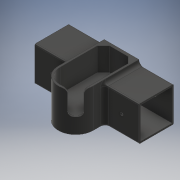
# Autodesk Inventor part: actuator_holder
Saved by Autodesk Inventor 2019.4 (Build 234330000, 330)
## iProperties
Created: 2020-10-05
Part Number: actuator_holder
Material: Generic
Document SubType Name: Modeling
Designer: deanv
Density: 1 g/cm^3
Appearance: Smooth - Black
Author: deanv
Autodesk Inventor part; units mm, degrees
ref_plane "YZ Plane" through (0, 0, 0) normal (1, 0, 0) x (0, 1, 0)
ref_plane "XZ Plane" through (0, 0, 0) normal (0, 1, 0) x (-1, 0, 0)
ref_plane "XY Plane" through (0, 0, 0) normal (0, 0, 1) x (1, 0, 0)
sketch "Sketch1" plane through (0, 0, 0) normal (0, 0, 1) x (1, 0, 0)
  line L0 (20, -37.4) -> (-20, -37.4) construction
  line L1 (-20, -37.4) -> (-20, 37.4) construction
  line L2 (-20, 37.4) -> (20, 37.4) construction
  line L3 (20, 37.4) -> (20, -37.4) construction
  line L4 (20, -37.4) -> (-20, 37.4) construction
  line L5 (-20, -37.4) -> (20, 37.4) construction
  line L6 (22.5, -39.9) -> (-22.5, -39.9) construction
  line L7 (-22.5, -39.9) -> (-22.5, 39.9) construction
  line L8 (-22.5, 39.9) -> (22.5, 39.9) construction
  line L9 (22.5, 39.9) -> (22.5, -39.9) construction
  line L10 (22.5, -39.9) -> (-22.5, 39.9) construction
  line L11 (-22.5, -39.9) -> (22.5, 39.9) construction
  line L12 (8.75, 10.75) -> (-8.75, 10.75)
  line L13 (-8.75, 10.75) -> (-8.75, 28.25)
  line L14 (-8.75, 28.25) -> (8.75, 28.25)
  line L15 (8.75, 28.25) -> (8.75, 10.75)
  line L16 (8.75, 10.75) -> (-8.75, 28.25) construction
  line L17 (-8.75, 10.75) -> (8.75, 28.25) construction
  line L18 (0, 39.9) -> (0, -39.9) construction
  line L19 (-22.5, 0) -> (22.5, 0) construction
  line L20 (-20, -17.4) -> (20, -17.4) construction
  line L21 (-20, 37.4) -> (20, 37.4)
  line L22 (20, 37.4) -> (20, -37.4)
  line L23 (20, -37.4) -> (-20, -37.4)
  line L24 (-20, -37.4) -> (-20, 37.4)
  line L25 (-22.5, -39.9) -> (22.5, -39.9)
  line L26 (22.5, -39.9) -> (22.5, 39.9)
  line L27 (22.5, 39.9) -> (-22.5, 39.9)
  line L28 (-22.5, 39.9) -> (-22.5, -39.9)
  line L29 (22.5, -0.5) -> (-22.5, -0.5) construction
  line L30 (-22.5, -0.5) -> (-22.5, 39.5) construction
  line L31 (-22.5, 39.5) -> (22.5, 39.5) construction
  line L32 (22.5, 39.5) -> (22.5, -0.5) construction
  line L33 (22.5, -0.5) -> (-22.5, 39.5) construction
  line L34 (-22.5, -0.5) -> (22.5, 39.5) construction
  line L35 (-22.5, 39.5) -> (22.5, 39.5)
  line L36 (22.5, 39.5) -> (22.5, 42)
  line L37 (22.5, 42) -> (-22.5, 42)
  line L38 (-22.5, 42) -> (-22.5, 39.5)
  line L39 (-22.5, -0.5) -> (22.5, -0.5)
  line L40 (22.5, -0.5) -> (22.5, -3)
  line L41 (22.5, -3) -> (-22.5, -3)
  line L42 (-22.5, -3) -> (-22.5, -0.5)
  line L43 (22.5, -39.9) -> (0, -17.4) construction
  line L44 (0, -39.9) -> (22.5, -17.4) construction
  line L45 (5.3033, -12.0967) -> (27.8033, -34.5967)
  line L46 (27.8033, -34.5967) -> (17.1967, -45.2033)
  line L47 (17.1967, -45.2033) -> (-5.3033, -22.7033)
  line L48 (-5.3033, -22.7033) -> (5.3033, -12.0967)
  line L49 (5.3033, -12.0967) -> (17.1967, -45.2033) construction
  line L50 (27.8033, -34.5967) -> (-5.3033, -22.7033) construction
  point P0 (0, 0)
  point P1 (0, 19.5)
  point P2 (0, 19.5)
  point P3 (11.25, -28.65)
  dimension "d0" = 40
  dimension "d1" = 74.8
  dimension "d2" = 79.8
  dimension "d3" = 45
  dimension "d4" = 17.5
  dimension "d5" = 17.5
  dimension "d6" = 20.4
  dimension "d7" = 20
  dimension "d12" = 40
  dimension "d13" = 2.5
  dimension "d14" = 2.5
  dimension "d78" = 22.5
  dimension "d79" = 15
  dimension "d80" = 22.5
  constraints: 102 end point, 20 parallel, 17 midpoint, 9 perpendicular, 8 horizontal, 6 point on line
  measures "d0" distance of L1.end L2.end
  measures "d1" distance of L0.end L1.end
  measures "d2" distance of L6.end L7.end
  measures "d3" distance of L7.end L8.end
  measures "d4" distance of L13.end L14.end
  measures "d5" distance between parallel lines of L14 L12
  measures "d6" distance from line of L8 point (0, 19.5)
  measures "d7" distance between parallel lines of L0 L20
  measures "d12" distance of L29.end L30.end
  measures "d13" distance of L36.end L35.end
  measures "d14" distance of L39.end L40.end
  measures "d78" horizontal distance of L18.end L44.end
  measures "d79" distance of L45.end L46.end
  measures "d80" horizontal distance of L45.start L45.end
extrude "Extrusion1" add sketch "Sketch1" along normal blind 20 contours L21 L22 L39 L24 | L39 L22 L41 L24 | L41 L22 L45 L48 L47 L23 L24 | L22 L23 L47 L48 L45
extrude "Extrusion2" add sketch "Sketch1" along normal blind 50 contours L24 L39 L28 L35 L26 L22 L21 | L24 L41 L28 L39 | L39 L26 L41 L22 | L24 L23 L47 L25 L28 L41 | L41 L26 L45 L22 | L28 L27 L26 L35 | L45 L26 L25 L47 L23 L22
extrude "Extrusion4" add sketch "Sketch1" along normal blind 50 contours L28 L27 L26 L35 | L38 L37 L36 L27
sketch "Sketch2" plane through (8.75, 10.75, 0) normal (-1, 0, 0) x (0, 0, 1)
  line L0 (0, 17.5) -> (20, 17.5) construction
  line L1 (20, 17.5) -> (20, 0) construction
  line L2 (20, 0) -> (0, 0) construction
  line L3 (0, 0) -> (0, 17.5) construction
  line L4 (20, 17.5) -> (10, 17.5) construction
  line L5 (10, 17.5) -> (10, 8.75) construction
  line L6 (10, 8.75) -> (20, 8.75) construction
  line L7 (20, 8.75) -> (20, 17.5) construction
  line L8 (10, 12.75) -> (10, 4.75) construction
  line L9 (6, 12.75) -> (6, 4.75)
  line L10 (14, 4.75) -> (14, 12.75)
  arc A0 (14, 12.75) -> (6, 12.75) centre (10, 12.75) ccw
  arc A1 (6, 4.75) -> (14, 4.75) centre (10, 4.75) ccw
  line L11 (10, 8.75) -> (18, 8.75) construction
  point P0 (0, -10.75)
  dimension "d19" = 10
  dimension "d20" = 8.75
  dimension "d96" = 4
  dimension "d97" = 90
  dimension "d98" = 8
  constraints: 26 end point, 5 parallel, 4 point on circle, 4 tangent, 3 horizontal, 3 perpendicular, 2 centre point, 1 coincident, 1 midpoint, 1 vertical
  measures "d19" distance of L6.end L5.end
  measures "d20" distance of L5.end L4.end
  measures "d96" distance of L11.start L8.end
  measures "d97" angle of L8 L11
  measures "d98" diameter of A1
fillet "Fillet1" radius 20 2 edges at (20, -37.4, 35) (-20, -37.4, 35)
fillet "Fillet2" radius 22.5 2 edges at (-22.5, -39.9, 25) (22.5, -39.9, 25)
sketch "Sketch4" plane through (22.5, 42, 50) normal (1, 0, 0) x (0, 0, -1)
  line L0 (50, 0) -> (0, 0) projected
  circle A0 centre (40, -22.5) radius 3 projected
  line L1 (30, -45) -> (50, -45) construction
  line L2 (50, -45) -> (50, 0) construction
  line L3 (50, 0) -> (30, 0) construction
  line L4 (30, 0) -> (30, -45) construction
  line L5 (30, -45) -> (50, 0) construction
  line L6 (50, -45) -> (30, 0) construction
  line L7 (50, -45) -> (5, -45)
  line L8 (5, -45) -> (5, 0)
  line L9 (5, 0) -> (50, 0)
  line L10 (50, 0) -> (50, -45)
  line L11 (5, -45) -> (50, 0) construction
  line L12 (50, -45) -> (5, 0) construction
  line L13 (48, -2) -> (7, -2)
  line L14 (7, -2) -> (7, -43)
  line L15 (7, -43) -> (48, -43)
  line L16 (48, -43) -> (48, -2)
  line L17 (48, -2) -> (7, -43) construction
  line L18 (7, -2) -> (48, -43) construction
  point P0 (50, -42)
  point P1 (27.5, -22.5)
  dimension "d42" = 45
  dimension "d43" = 45
  dimension "d44" = 41
  dimension "d45" = 41
  constraints: 36 end point, 6 parallel, 5 midpoint, 3 horizontal, 3 perpendicular, 1 point on line
  measures "d42" distance of L0.start L1.end
  measures "d43" distance of L8.end L9.end
  measures "d44" distance of L15.end L14.end
  measures "d45" distance of L14.end L13.end
extrude "Extrusion5" add sketch "Sketch4" along normal blind 45 contours L10 L7 L8 L0
sketch "Sketch6" plane through (-22.5, 42, 0) normal (-1, 0, 0) x (0, 0, 1)
  line L0 (0, 0) -> (45, 0)
  line L1 (45, 0) -> (45, -45)
  line L2 (45, -45) -> (0, -45)
  line L3 (0, -45) -> (0, 0)
  line L4 (2, -43) -> (43, -43)
  line L5 (43, -43) -> (43, -2)
  line L6 (43, -2) -> (2, -2)
  line L7 (2, -2) -> (2, -43)
  line L8 (2, -43) -> (43, -2) construction
  line L9 (43, -43) -> (2, -2) construction
  point P0 (0, -42)
  point P1 (22.5, -22.5)
  dimension "d53" = 45
  dimension "d54" = 45
  dimension "d55" = 41
  dimension "d56" = 41
  dimension "d57" = 2
  dimension "d58" = 2
  constraints: 20 end point, 4 parallel, 2 horizontal, 2 midpoint, 2 perpendicular
  measures "d53" distance of L1.end L2.end
  measures "d54" distance of L0.end L1.end
  measures "d55" distance of L4.end L5.end
  measures "d56" distance of L5.end L6.end
  measures "d57" distance between parallel lines of L1 L5
  measures "d58" distance between parallel lines of L0 L6
extrude "Extrusion6" add sketch "Sketch6" along normal blind 45
fillet "Fillet5" radius 1.5 7 edges at (45, -3, 45) (45, 42, 45) (45, -3, 0) (0, 42, 0) (-45, -3, 45) (-45, 42, 45) (-45, -3, 0)
fillet "Fillet6" radius 5 10 edges at (22.5, 41.5607, 44.5607) (22.5, -2.5607, 44.5607) (22.5, -3, 22.5) (22.5, -2.5607, 0.4393) (22.5, 19.5, 45) (-22.5, -2.5607, 44.5607) (-22.5, -3, 22.5) (-22.5, -2.5607, 0.4393) (-22.5, 41.5607, 44.5607) (-22.5, 19.5, 45)
sketch "Sketch7" plane through (-22.5, 42, 50) normal (0, 1, 0) x (1, 0, 0)
  line L0 (-45, 5) -> (-45, 6.5) construction
  line L1 (90, 50) -> (-45, 50) construction
  line L2 (-45, 50) -> (-45, 5) construction
  line L3 (-45, 5) -> (90, 5) construction
  line L4 (90, 5) -> (90, 50) construction
  line L5 (90, 5) -> (45, 5) construction
  line L6 (45, 5) -> (45, 50) construction
  line L7 (45, 50) -> (90, 50) construction
  line L8 (90, 50) -> (90, 5) construction
  line L9 (-45, 5) -> (0, 5) construction
  line L10 (0, 5) -> (0, 50) construction
  line L11 (0, 50) -> (-45, 50) construction
  line L12 (-45, 50) -> (-45, 5) construction
  line L13 (90, 6.5) -> (90, 5) construction
  line L14 (90, 5) -> (45, 50) construction
  line L15 (0, 50) -> (-45, 5) construction
  line L16 (-45, 50) -> (0, 5) construction
  line L17 (90, 50) -> (45, 5) construction
  circle A0 centre (67.5, 27.5) radius 2
  circle A1 centre (-22.5, 27.5) radius 2
  point P0 (22.5, 50)
  dimension "d63" = 45
  dimension "d64" = 45
  dimension "d65" = 45
  dimension "d66" = 45
  dimension "d74" = 4
  dimension "d75" = 4
  constraints: 32 end point, 6 parallel, 3 horizontal, 3 perpendicular, 2 centre point, 2 coincident, 2 midpoint
  measures "d63" distance of L6.end L7.end
  measures "d64" distance of L5.end L6.end
  measures "d65" distance of L11.end L10.end
  measures "d66" distance of L10.end L9.end
  measures "d74" diameter of A0
  measures "d75" diameter of A1
extrude "Extrusion7" cut sketch "Sketch7" against normal blind 45
sketch "Sketch8" plane through (0, 0, 50) normal (0, 0, 1) x (1, 0, 0)
  arc A0 (-20, -17.4) -> (20, -17.4) centre (0, -17.4) ccw projected
  line L0 (0, -17.4) -> (22.5, -17.4) construction
  line L1 (22.5, -17.4) -> (22.5, -39.9) construction
  line L2 (22.5, -39.9) -> (0, -39.9) construction
  line L3 (0, -39.9) -> (0, -17.4) construction
  line L4 (22.5, -39.9) -> (0, -17.4) construction
  line L5 (22.5, -17.4) -> (0, -39.9) construction
  line L6 (27.8033, -34.5967) -> (5.3033, -12.0967)
  line L7 (5.3033, -12.0967) -> (-5.3033, -22.7033)
  line L8 (-5.3033, -22.7033) -> (17.1967, -45.2033)
  line L9 (17.1967, -45.2033) -> (27.8033, -34.5967)
  line L10 (27.8033, -34.5967) -> (-5.3033, -22.7033) construction
  line L11 (5.3033, -12.0967) -> (17.1967, -45.2033) construction
  line L12 (22.5, -1.5) -> (22.5, 40.5) projected
  line L13 (22.5, 42) -> (-22.5, 42) projected
  line L14 (-22.5, 42) -> (22.5, 42) construction
  line L15 (22.5, 42) -> (22.5, 0) construction
  line L16 (22.5, 0) -> (-22.5, 0) construction
  line L17 (-22.5, 0) -> (-22.5, 42) construction
  line L18 (-20, 29.4) -> (20, 29.4)
  line L19 (20, 29.4) -> (20, 38.4)
  line L20 (20, 38.4) -> (-20, 38.4)
  line L21 (-20, 38.4) -> (-20, 29.4)
  point P0 (0, 0)
  point P1 (11.25, -28.65)
  dimension "d81" = 22.5
  dimension "d82" = 22.5
  dimension "d83" = 15
  dimension "d84" = 31.8198
  dimension "d88" = 42
  dimension "d89" = 40
  dimension "d90" = 9
  constraints: 40 end point, 9 parallel, 4 perpendicular, 3 horizontal, 3 midpoint, 1 point on line
  measures "d81" distance of L0.end L1.end
  measures "d82" distance of L1.end L2.end
  measures "d83" distance of L7.end L6.end
  measures "d84" distance between parallel lines of L7 L9
  measures "d88" distance between parallel lines of L13 L16
  measures "d89" distance of L20.end L19.end
  measures "d90" distance of L19.end L18.end
extrude "Extrusion8" cut sketch "Sketch8" against normal blind 30 contours L8 L7 L6 A0 | A0 L6 L9 L8
fillet "Fillet7" radius 5 4 edges at (8.7518, -36.7584, 50) (19.3584, -26.1518, 50) (8.7518, -36.7584, 20) (19.3584, -26.1518, 20)
extrude "Extrusion9" cut sketch "Sketch8" against normal blind 30 contours L21 L20 L19 L18
chamfer "Chamfer2" distance 8 angle 45 2 edges at (-20, 38.4, 35) (20, 38.4, 35)
extrude "Extrusion10" cut sketch "Sketch2" along normal mid plane 75
equation "\"d5\" = d4"
equation "\"d56\" = d55"
equation "\"d57\" = 0.5 * d53 - 0.5 * d56"
equation "\"d58\" = d57"
body "Solid1"
